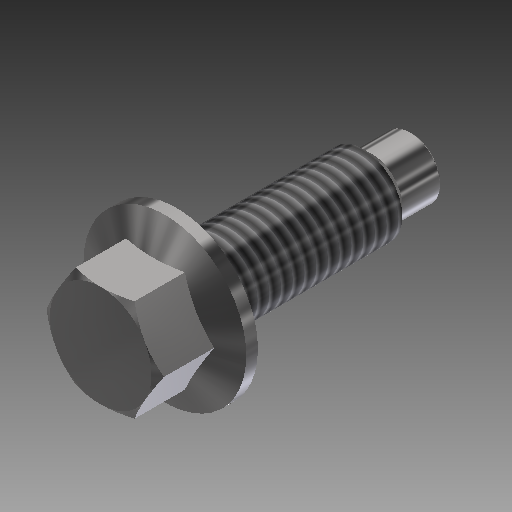
# Autodesk Inventor part: 202-10
Saved by Autodesk Inventor 2019 (Build 230136000, 136)
## iProperties
Company: Autodesk Inc.
Created: 2007-11-01
Part Number: 202-10
Document SubType Name: Modeling
Designer: Autodesk Inc.
Density: 8 g/cm^3
Mass: 32.1477 g
Surface Area: 19.7101 cm^2
Volume: 4.01847 cm^3
Material: Stainless Steel
Description: H343 BOLT M12 X 20
Appearance: Semi-Polished
Component Category: Fasteners
Author: Inventor
Autodesk Inventor part; units mm, degrees
ref_plane "YZ Plane" through (0, 0, 0) normal (1, 0, 0) x (0, 1, 0)
ref_plane "XZ Plane" through (0, 0, 0) normal (0, 1, 0) x (-1, 0, 0)
ref_plane "XY Plane" through (0, 0, 0) normal (0, 0, 1) x (1, 0, 0)
sketch "Sketch1" plane through (0, 0, 0) normal (0, 0, 1) x (1, 0, 0)
  line L0 (-10.5078, 0) -> (10.5078, 0) projected
  line L1 (7.5056, 0) -> (3.7528, -6.5)
  line L2 (3.7528, -6.5) -> (-3.7528, -6.5)
  line L3 (-3.7528, -6.5) -> (-7.5056, 0)
  line L4 (-7.5056, 0) -> (-3.7528, 6.5)
  line L5 (-3.7528, 6.5) -> (3.7528, 6.5)
  line L6 (3.7528, 6.5) -> (7.5056, 0)
  point P0 (0, 0)
  point P1 (0, 0)
  dimension "d0" = 13
  constraints: 12 end point, 1 coincident, 1 point on line, 13 other
  measures "d0" distance between parallel lines of L2 L5
extrude "Extrusion1" add sketch "Sketch1" against normal blind 9.7
sketch "Sketch2" plane through (0, 0, 0) normal (0, 1, 0) x (-1, 0, 0)
  line L0 (3.7528, -9.7) -> (-3.7528, -9.7) projected
  line L1 (7.5056, -9.7) -> (3.7528, -9.7) projected
  line L2 (3.7528, -9.7) -> (7.5056, -9.7) projected
  line L3 (-3.7528, -9.7) -> (3.7528, -9.7) projected
  line L4 (-7.5056, -9.7) -> (-3.7528, -9.7) projected
  line L5 (-3.7528, -9.7) -> (-7.5056, -9.7) projected
  line L6 (0, -9.7) -> (-10.4, -9.7)
  line L7 (-10.4, -9.7) -> (-10.4, -8.2)
  line L8 (-10.4, -8.2) -> (0, -3.8922)
  line L9 (0, -3.8922) -> (0, -9.7)
  line L10 (-5, -9.7) -> (-5, -33.55)
  line L11 (-5, -33.55) -> (-3.85, -34.7)
  line L12 (-3.85, -34.7) -> (-3.85, -39.7)
  line L13 (-3.85, -39.7) -> (0, -39.7)
  line L14 (0, -9.7) -> (0, -39.7)
  point P0 (0, 0)
  dimension "d3" = 1.5
  dimension "d4" = 10.4
  dimension "d5" = 22.5
  dimension "d7" = 5
  dimension "d8" = 3.85
  dimension "d9" = 30
  dimension "d10" = 5
  dimension "d11" = 1.15
  constraints: 18 end point, 4 perpendicular, 2 parallel, 2 point on line, 1 midpoint
  measures "d3" distance of L6.end L7.end
  measures "d4" distance of L6.start L6.end
  measures "d5" angle of L6 L8
  measures "d7" distance between parallel lines of L14 L10
  measures "d8" distance between parallel lines of L14 L12
  measures "d9" distance between parallel lines of L6 L13
  measures "d10" distance from line of L11.end L13
  measures "d11" horizontal distance of L10.end L11.end
revolve "Revolution1" add sketch "Sketch2" angle 360 about axis through (0, 0, -9.7) along (0, 0, -1)
sketch "Sketch3" plane through (0, 0, 0) normal (0, 1, 0) x (-1, 0, 0)
  line L0 (-6.5, 0) -> (-7.5056, -0.5806)
  line L1 (-7.5056, -0.5806) -> (-7.5056, 0)
  line L2 (-7.5056, 0) -> (-6.5, 0)
  line L3 (0, -0.6967) -> (0, 0.1161) projected
  point P0 (0, 0)
  dimension "d13" = 30
  dimension "d14" = 1.0055
  dimension "d16" = 6.5
  constraints: 6 end point, 1 perpendicular, 1 point on line, 1 vertical
  measures "d13" angle of L0 L2
  measures "d14" distance of L1.end L0.start
  measures "d16" distance of L0.start point (0, 0)
revolve "Revolution2" cut sketch "Sketch3" angle 360 about axis through (0, 0, 0) along (0, 0, 1)
thread "Thread1" size "M10x1.5" class "6g" standard "ANSI Metric M Profile" full length
fillet "Fillet1" radius 0.2 1 edges at (-3.85, 0, -39.7)
body "Solid1"
